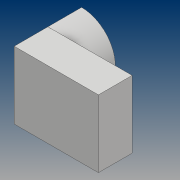
# Autodesk Inventor part: 39 (60283.185 mm^3)
Saved by Autodesk Inventor 2018 (Build 220112000, 112)
## iProperties
Created: 2020-09-18
Part Number: 39 (60283.185 mm^3)
Material: 一般
Document SubType Name: Modeling
Designer: 88697
Density: 1 g/cm^3
Appearance: 預設
Author: 88697
Autodesk Inventor part; units mm, degrees
ref_plane "YZ Plane" through (0, 0, 0) normal (1, 0, 0) x (0, 1, 0)
ref_plane "XZ Plane" through (0, 0, 0) normal (0, 1, 0) x (-1, 0, 0)
ref_plane "XY Plane" through (0, 0, 0) normal (0, 0, 1) x (1, 0, 0)
sketch "草圖1" plane through (0, 0, 0) normal (0, 1, 0) x (-1, 0, 0)
  line L0 (0, 0) -> (-50, 0)
  line L1 (-50, 0) -> (-50, -40)
  line L2 (-50, -40) -> (0, -40)
  line L3 (0, -40) -> (0, 0)
  dimension "d0" = 50
  dimension "d1" = 40
  constraints: 8 end point, 2 parallel, 1 horizontal, 1 perpendicular
  measures "d0" distance of L0.start L0.end
  measures "d1" distance of L2.end L0.start
extrude "擠出1" add sketch "草圖1" along normal blind 20
sketch "草圖2" plane through (0, 20, 0) normal (0, 1, 0) x (1, 0, 0)
  line L0 (0, 40) -> (20, 40)
  line L1 (20, 40) -> (20, 0)
  line L2 (20, 0) -> (0, 0)
  line L3 (0, 0) -> (0, 40)
  line L4 (50, 40) -> (0, 40) projected
  line L5 (0, 40) -> (0, 0) projected
  dimension "d4" = 20
  constraints: 8 end point, 2 collinear, 2 parallel, 1 horizontal, 1 perpendicular
  measures "d4" distance between parallel lines of L3 L1
extrude "擠出2" add sketch "草圖2" along normal blind 20
fillet "圓角1" radius 20 1 edges at (20, 30, 0)
sketch "草圖3" plane through (50, 0, -40) normal (0, 0, -1) x (-1, 0, 0)
  line L0 (30, 40) -> (50, 40) projected
  line L1 (0, 20) -> (30, 20) projected
  line L2 (30, 40) -> (0, 20)
  line L3 (0, 20) -> (30, 20)
  line L4 (30, 20) -> (30, 40) projected
  line L5 (30, 20) -> (30, 40)
  point P0 (50, 0)
  constraints: 6 end point, 2 collinear
extrude "擠出3" add sketch "草圖3" against normal blind 20
